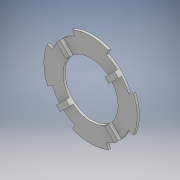
# Autodesk Inventor part: Dome Clip
Saved by Autodesk Inventor 2017 (Build 210142000, 142)
## iProperties
Created: 2018-02-14
Part Number: Dome Clip
Material: Generic
Document SubType Name: Modeling
Designer: Arjuna
Density: 1 g/cm^3
Appearance: Default
Author: Arjuna
## iProperties of the stored document Dome Clip_3DPrint.ipt
Created: 2018-03-29
Part Number: Dome Clip_3DPrint
Material: Generic
Document SubType Name: Modeling
Designer: Arjuna
Density: 1 g/cm^3
Appearance: Default
Author: Arjuna
Autodesk Inventor part; units mm, degrees
ref_plane "YZ Plane" through (0, 0, 0) normal (1, 0, 0) x (0, 1, 0)
ref_plane "XZ Plane" through (0, 0, 0) normal (0, 1, 0) x (-1, 0, 0)
ref_plane "XY Plane" through (0, 0, 0) normal (0, 0, 1) x (1, 0, 0)
sketch "Sketch1" plane through (0, 0, 0) normal (0, 1, 0) x (-1, 0, 0)
  circle A0 centre (0, 0) radius 42.75
  circle A1 centre (0, 0) radius 25.25
  dimension "d0" = 85.5
  dimension "d1" = 50.5
  constraints: 2 centre point, 2 coincident
  measures "d0" diameter of A0
  measures "d1" diameter of A1
extrude "Extrusion1" add sketch "Sketch1" along normal blind 2
sketch "Sketch2" plane through (0, 2, 0) normal (0, 1, 0) x (1, 0, 0)
  circle A0 centre (0, 0) radius 25.25 projected
  circle A1 centre (0, 0) radius 42.75 projected
  line L0 (0, 0) -> (26.6933, 26.6933)
  arc A2 (39.4959, 16.3597) -> (30.2288, 30.2288) centre (0, 0) ccw
  line L1 (0, 0) -> (39.4959, 16.3597) construction
  line L2 (0, 0) -> (26.6933, 26.6933) construction
  arc A3 (30.2288, 30.2288) -> (16.3597, 39.4959) centre (0, 0) ccw
  line L3 (0, 0) -> (30.2288, 30.2288) construction
  line L4 (0, 0) -> (17.5537, 7.271) construction
  line L5 (0, 0) -> (17.8544, 17.8544) construction
  line L6 (0, 0) -> (9.6628, 23.328) construction
  line L7 (0, 0) -> (17.8544, 17.8544) construction
  line L8 (16.3597, 39.4959) -> (14.4463, 34.8765)
  line L9 (34.8765, 14.4463) -> (39.4959, 16.3597)
  arc A4 (34.8765, 14.4463) -> (14.4463, 34.8765) centre (0, 0) ccw
  line L10 (16.3597, 39.4959) -> (14.4463, 34.8765)
  line L11 (39.4959, 16.3597) -> (34.8765, 14.4463)
  line L12 (0, 0) -> (9.6628, 23.328) construction
  line L13 (14.4463, 34.8765) -> (16.3597, 39.4959) construction
  line L14 (-39.4959, 16.3597) -> (-34.8765, 14.4463)
  arc A5 (-30.2288, 30.2288) -> (-39.4959, 16.3597) centre (0, 0) ccw
  arc A6 (-16.3597, 39.4959) -> (-30.2288, 30.2288) centre (0, 0) ccw
  line L15 (-14.4463, 34.8765) -> (-16.3597, 39.4959)
  arc A7 (-14.4463, 34.8765) -> (-34.8765, 14.4463) centre (0, 0) ccw
  line L16 (-16.3597, -39.4959) -> (-14.4463, -34.8765)
  arc A8 (-30.2288, -30.2288) -> (-16.3597, -39.4959) centre (0, 0) ccw
  arc A9 (-39.4959, -16.3597) -> (-30.2288, -30.2288) centre (0, 0) ccw
  line L17 (-34.8765, -14.4463) -> (-39.4959, -16.3597)
  arc A10 (-34.8765, -14.4463) -> (-14.4463, -34.8765) centre (0, 0) ccw
  line L18 (39.4959, -16.3597) -> (34.8765, -14.4463)
  arc A11 (30.2288, -30.2288) -> (39.4959, -16.3597) centre (0, 0) ccw
  arc A12 (16.3597, -39.4959) -> (30.2288, -30.2288) centre (0, 0) ccw
  line L19 (14.4463, -34.8765) -> (16.3597, -39.4959)
  arc A13 (14.4463, -34.8765) -> (34.8765, -14.4463) centre (0, 0) ccw
  point P0 (-26.6933, 26.6933)
  point P1 (-26.6933, -26.6933)
  point P2 (26.6933, -26.6933)
  dimension "d4" = 22.5
  dimension "d8" = 75.5
  dimension "d11" = 360
  constraints: 40 end point, 32 point on circle, 12 centre point, 8 coincident, 2 point on line, 57 other
  measures "d4" angle of L1 L2
  measures "d8" diameter of A4
extrude "Extrusion2" cut sketch "Sketch2" against normal through all contours A4 L8 A1 L9 | L15 A7 L14 A1 | A1 L19 A13 L18 | L17 A10 L16 A1
sketch "Sketch5" plane through (0, 0, 0) normal (0, -1, 0) x (1, 0, 0)
  line L0 (-16.3597, 39.4959) -> (-14.4463, 34.8765) projected
  line L1 (-34.8765, 14.4463) -> (-39.4959, 16.3597) projected
  arc A0 (-39.4959, 16.3597) -> (-39.4959, -16.3597) centre (0, 0) ccw projected
  line L2 (-39.4959, -16.3597) -> (-34.8765, -14.4463) projected
  line L3 (-14.4463, -34.8765) -> (-16.3597, -39.4959) projected
  arc A1 (-16.3597, -39.4959) -> (16.3597, -39.4959) centre (0, 0) ccw projected
  line L4 (16.3597, -39.4959) -> (14.4463, -34.8765) projected
  line L5 (34.8765, -14.4463) -> (39.4959, -16.3597) projected
  arc A2 (39.4959, -16.3597) -> (39.4959, 16.3597) centre (0, 0) ccw projected
  line L6 (39.4959, 16.3597) -> (34.8765, 14.4463) projected
  line L7 (14.4463, 34.8765) -> (16.3597, 39.4959) projected
  arc A3 (16.3597, 39.4959) -> (-16.3597, 39.4959) centre (0, 0) ccw projected
  circle A4 centre (0, 0) radius 25.25 projected
  line L8 (0, 0) -> (-17.8544, -17.8544)
  line L9 (0, 0) -> (-5.6762, 0)
  line L10 (-19.8816, -22.7984) -> (-16.3892, -19.2083)
  line L11 (-22.8427, -19.8307) -> (-19.2083, -16.3892)
  arc A5 (-19.2083, -16.3892) -> (-16.3892, -19.2083) centre (0, 0) ccw
  arc A6 (-22.8427, -19.8307) -> (-19.8816, -22.7984) centre (0, 0) ccw
  line L12 (22.7984, -19.8816) -> (19.2083, -16.3892)
  line L13 (19.8307, -22.8427) -> (16.3892, -19.2083)
  arc A7 (16.3892, -19.2083) -> (19.2083, -16.3892) centre (0, 0) ccw
  arc A8 (19.8307, -22.8427) -> (22.7984, -19.8816) centre (0, 0) ccw
  line L14 (19.8816, 22.7984) -> (16.3892, 19.2083)
  line L15 (22.8427, 19.8307) -> (19.2083, 16.3892)
  arc A9 (19.2083, 16.3892) -> (16.3892, 19.2083) centre (0, 0) ccw
  arc A10 (22.8427, 19.8307) -> (19.8816, 22.7984) centre (0, 0) ccw
  line L16 (-22.7984, 19.8816) -> (-19.2083, 16.3892)
  line L17 (-19.8307, 22.8427) -> (-16.3892, 19.2083)
  arc A11 (-16.3892, 19.2083) -> (-19.2083, 16.3892) centre (0, 0) ccw
  arc A12 (-19.8307, 22.8427) -> (-22.7984, 19.8816) centre (0, 0) ccw
  arc A13 (-14.4463, 34.8765) -> (-34.8765, 14.4463) centre (0, 0) ccw projected
  arc A14 (-34.8765, -14.4463) -> (-14.4463, -34.8765) centre (0, 0) ccw projected
  arc A15 (14.4463, -34.8765) -> (34.8765, -14.4463) centre (0, 0) ccw projected
  arc A16 (34.8765, 14.4463) -> (14.4463, 34.8765) centre (0, 0) ccw projected
  point P0 (17.8544, -17.8544)
  point P1 (17.8544, 17.8544)
  point P2 (-17.8544, 17.8544)
  dimension "d31" = 45
  dimension "d35" = 360
  constraints: 20 end point, 20 point on circle, 8 centre point, 2 coincident, 1 horizontal, 47 other
  measures "d31" angle of L8 L9
extrude "Extrusion4" [suppressed]
sketch "Sketch6" plane through (0, 0, 0) normal (0, -1, 0) x (1, 0, 0)
  line L0 (-16.3597, 39.4959) -> (-14.4463, 34.8765) projected
  arc A0 (-14.4463, 34.8765) -> (-34.8765, 14.4463) centre (0, 0) ccw projected
  line L1 (-34.8765, 14.4463) -> (-39.4959, 16.3597) projected
  arc A1 (-39.4959, 16.3597) -> (-39.4959, -16.3597) centre (0, 0) ccw projected
  line L2 (-39.4959, -16.3597) -> (-34.8765, -14.4463) projected
  arc A2 (-34.8765, -14.4463) -> (-14.4463, -34.8765) centre (0, 0) ccw projected
  line L3 (-14.4463, -34.8765) -> (-16.3597, -39.4959) projected
  arc A3 (-16.3597, -39.4959) -> (16.3597, -39.4959) centre (0, 0) ccw projected
  line L4 (16.3597, -39.4959) -> (14.4463, -34.8765) projected
  arc A4 (14.4463, -34.8765) -> (34.8765, -14.4463) centre (0, 0) ccw projected
  line L5 (34.8765, -14.4463) -> (39.4959, -16.3597) projected
  arc A5 (39.4959, -16.3597) -> (39.4959, 16.3597) centre (0, 0) ccw projected
  line L6 (39.4959, 16.3597) -> (34.8765, 14.4463) projected
  arc A6 (34.8765, 14.4463) -> (14.4463, 34.8765) centre (0, 0) ccw projected
  line L7 (14.4463, 34.8765) -> (16.3597, 39.4959) projected
  arc A7 (16.3597, 39.4959) -> (-16.3597, 39.4959) centre (0, 0) ccw projected
  circle A8 centre (0, 0) radius 25.25 projected
  line L8 (0, 0) -> (26.6933, 26.6933)
  line L9 (15.999, 19.5345) -> (19.5345, 15.999)
  arc A9 (19.5345, 15.999) -> (15.999, 19.5345) centre (0, 0) ccw
  line L10 (19.5345, 15.999) -> (28.4024, 24.8669)
  line L11 (15.999, 19.5345) -> (24.8669, 28.4024)
  arc A10 (28.4024, 24.8669) -> (24.8669, 28.4024) centre (0, 0) ccw
  line L12 (-19.5345, 15.999) -> (-15.999, 19.5345)
  arc A11 (-15.999, 19.5345) -> (-19.5345, 15.999) centre (0, 0) ccw
  line L13 (-15.999, 19.5345) -> (-24.8669, 28.4024)
  line L14 (-19.5345, 15.999) -> (-28.4024, 24.8669)
  arc A12 (-24.8669, 28.4024) -> (-28.4024, 24.8669) centre (0, 0) ccw
  line L15 (-15.999, -19.5345) -> (-19.5345, -15.999)
  arc A13 (-19.5345, -15.999) -> (-15.999, -19.5345) centre (0, 0) ccw
  line L16 (-19.5345, -15.999) -> (-28.4024, -24.8669)
  line L17 (-15.999, -19.5345) -> (-24.8669, -28.4024)
  arc A14 (-28.4024, -24.8669) -> (-24.8669, -28.4024) centre (0, 0) ccw
  line L18 (19.5345, -15.999) -> (15.999, -19.5345)
  arc A15 (15.999, -19.5345) -> (19.5345, -15.999) centre (0, 0) ccw
  line L19 (15.999, -19.5345) -> (24.8669, -28.4024)
  line L20 (19.5345, -15.999) -> (28.4024, -24.8669)
  arc A16 (24.8669, -28.4024) -> (28.4024, -24.8669) centre (0, 0) ccw
  point P0 (-26.6933, 26.6933)
  point P1 (-26.6933, -26.6933)
  point P2 (26.6933, -26.6933)
  dimension "d39" = 5
  dimension "d40" = 2.5
  dimension "d43" = 360
  constraints: 26 end point, 21 point on circle, 8 centre point, 5 coincident, 1 parallel, 1 perpendicular, 49 other
  measures "d39" distance of L9.start L9.end
  measures "d40" distance from line of L8 L9.start
extrude "Extrusion5" add sketch "Sketch6" along normal blind 3 contours L13 A8 L14 A0 | A6 L8 A8 L11 | A6 L10 A8 L8 | A8 L17 A2 L16 | A8 L20 A4 L19
equation "\"d40\" = 0.5 * d39"
body "Solid1"
